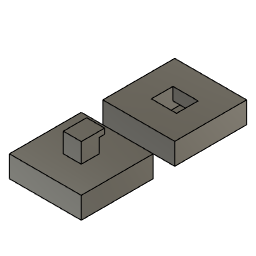
Latch cube 1 v2 (Autodesk Fusion 360 design; units mm, degrees)
Autodesk Fusion 360 part; units mm, degrees
sketch "Sketch1" plane through (0, 0, 0) normal (0, 0, 1) x (1, 0, 0) in component "Out put"
  line L0 (10, -10) -> (-10, -10)
  line L1 (-10, -10) -> (-10, 10)
  line L2 (-10, 10) -> (10, 10)
  line L3 (10, 10) -> (10, -10)
  line L4 (10, -10) -> (-10, 10) construction
  line L5 (-10, -10) -> (10, 10) construction
  dimension "d1" = 20
  dimension "d2" = 20
  constraint horizontal L0
  constraint perpendicular L0 L1
  constraint parallel L0 L2
  constraint parallel L1 L3
  constraint coincident L4 origin
  constraint coincident L5 origin
  measures "d1" distance of L1.end L2.end
  measures "d2" distance of L0.end L1.end
extrude "Extrude1" add sketch "Sketch1" along normal blind 6 makes body 1 in component "Out put"
sketch "Sketch2" plane through (0, 0, 6) normal (0, 0, 1) x (-1, 0, 0) in component "Out put"
  line L0 (-10, -10) -> (10, -10)
  line L1 (10, -10) -> (10, 10)
  line L2 (10, 10) -> (-10, 10)
  line L3 (-10, 10) -> (-10, -10)
  line L4 (-2.5, 2.5) -> (2.5, 2.5)
  line L5 (2.5, 2.5) -> (2.5, -2.5)
  line L6 (2.5, -2.5) -> (-2.5, -2.5)
  line L7 (-2.5, -2.5) -> (-2.5, 2.5)
  line L8 (-2.5, 2.5) -> (2.5, -2.5) construction
  line L9 (2.5, 2.5) -> (-2.5, -2.5) construction
  dimension "d5" = 5
  dimension "d6" = 5
  constraint horizontal L4
  constraint perpendicular L4 L5
  constraint parallel L4 L6
  constraint parallel L5 L7
  constraint coincident L8 origin
  constraint coincident L9 origin
  measures "d5" distance of L5.end L6.end
  measures "d6" distance of L4.end L5.end
extrude "Extrude2" add sketch "Sketch2" along normal blind 5.45 contours L4 L5 L6 L7 bodies 1 in component "Out put"
sketch "Sketch3" plane through (0, 2.5, 0) normal (0, 1, 0) x (-1, 0, 0) in component "Out put"
  line L0 (-2.5, 6) -> (2.5, 6)
  line L1 (2.5, 6) -> (2.5, 11.45)
  line L2 (2.5, 11.45) -> (-2.5, 11.45)
  line L3 (-2.5, 11.45) -> (-2.5, 6)
  line L4 (-2.5, 11.45) -> (2.5, 11.45)
  line L5 (2.5, 11.45) -> (2.5, 9.95)
  line L6 (2.5, 9.95) -> (-2.5, 9.95)
  line L7 (-2.5, 9.95) -> (-2.5, 11.45)
  dimension "d9" = 5
  dimension "d10" = 1.5
  constraint horizontal L4
  constraint vertical L5
  constraint horizontal L6
  constraint vertical L7
  constraint coincident L2.end L3.start
  measures "d9" distance of L2.end L1.end
  measures "d10" distance of L2.end L6.end
extrude "Extrude3" add sketch "Sketch3" along normal blind 1.5 contours L1 L2 L3 L4 L5 L6 L7 bodies 1 in component "Out put"
move_body "Move1" bodies 1 to x (1, 0, 0) y (0, 1, 0) z (0, 0, 1) at (0, -30, 0) in component "Out put"
sketch "Sketch1 (2)" plane through (0, 0, 0) normal (0, 0, 1) x (1, 0, 0) in component "Input"
  line L0 (-10, 10) -> (10, 10)
  line L1 (10, 10) -> (10, -10)
  line L2 (10, -10) -> (-10, -10)
  line L3 (-10, -10) -> (-10, 10)
  line L4 (-10, 10) -> (10, -10) construction
  line L5 (10, 10) -> (-10, -10) construction
  dimension "d13" = 20
  dimension "d14" = 20
  constraint horizontal L0
  constraint perpendicular L0 L1
  constraint parallel L0 L2
  constraint parallel L1 L3
  constraint coincident L4 origin
  constraint coincident L5 origin
  measures "d13" distance of L1.end L2.end
  measures "d14" distance of L0.end L1.end
extrude "Extrude1'" add sketch "Sketch1 (2)" along normal blind 6 separate body makes body 2 in component "Input"
sketch "Sketch3 (2)" plane through (0, 0, 6) normal (0, 0, 1) x (-1, 0, 0) in component "Input"
  line L0 (10, 10) -> (-10, 10)
  line L1 (-10, 10) -> (-10, -10)
  line L2 (-10, -10) -> (10, -10)
  line L3 (10, -10) -> (10, 10)
  line L4 (-3.5, 3) -> (3.5, 3)
  line L5 (3.5, 3) -> (3.5, -3)
  line L6 (3.5, -3) -> (-3.5, -3)
  line L7 (-3.5, -3) -> (-3.5, 3)
  line L8 (-3.5, 3) -> (3.5, -3) construction
  line L9 (3.5, 3) -> (-3.5, -3) construction
  dimension "d21" = 7
  dimension "d22" = 6
  constraint horizontal L4
  constraint perpendicular L4 L5
  constraint parallel L4 L6
  constraint parallel L5 L7
  constraint coincident L8 origin
  constraint coincident L9 origin
  measures "d21" distance of L5.end L6.end
  measures "d22" distance of L4.end L5.end
extrude "Extrude3'" cut sketch "Sketch3 (2)" against normal blind 5.5 contours L4 L5 L6 L7 bodies 2 in component "Input"
sketch "Sketch4" plane through (0, 3, 0) normal (0, -1, 0) x (1, 0, 0) in component "Input"
  line L0 (3.5, 6) -> (-3.5, 6)
  line L1 (-3.5, 6) -> (-3.5, 0.5)
  line L2 (-3.5, 0.5) -> (3.5, 0.5)
  line L3 (3.5, 0.5) -> (3.5, 6)
  line L4 (-3.5, 0.5) -> (3.5, 0.5)
  line L5 (3.5, 0.5) -> (3.5, 2.5)
  line L6 (3.5, 2.5) -> (-3.5, 2.5)
  line L7 (-3.5, 2.5) -> (-3.5, 0.5)
  dimension "d25" = 7
  dimension "d26" = 2
  constraint horizontal L4
  constraint vertical L5
  constraint horizontal L6
  constraint vertical L7
  constraint coincident L1.end L2.start
  measures "d25" distance of L1.end L2.end
  measures "d26" distance of L1.end L6.end
extrude "Extrude4" cut sketch "Sketch4" against normal blind 2 contours L1 L2 L3 L4 L5 L6 L7 bodies 2 in component "Input"
sketch "Sketch5" plane through (3.5, 0, 0) normal (-1, 0, 0) x (0, -1, 0) in component "Input"
  line L0 (3, 6) -> (-3, 6)
  line L1 (-3, 6) -> (-3, 2.5)
  line L2 (-3, 2.5) -> (-5, 2.5)
  line L3 (-5, 2.5) -> (-5, 0.5)
  line L4 (-5, 0.5) -> (3, 0.5)
  line L5 (3, 0.5) -> (3, 6)
  line L6 (-5, 0.5) -> (3, 0.5)
  line L7 (3, 0.5) -> (3, 2.5)
  line L8 (3, 2.5) -> (-5, 2.5)
  line L9 (-5, 2.5) -> (-5, 0.5)
  dimension "d29" = 8
  dimension "d30" = 2
  constraint horizontal L6
  constraint vertical L7
  constraint horizontal L8
  constraint vertical L9
  constraint coincident L3.end L4.start
  measures "d29" distance of L3.end L4.end
  measures "d30" distance of L3.end L2.end
extrude "Extrude5" cut sketch "Sketch5" against normal blind 2 contours L2 L3 L4 L5 L6 L7 L8 L9 bodies 2 in component "Input"
move_body "Move1'" bodies 2 to x (1, 0, 0) y (0, 1, 0) z (0, 0, 1) at (0, 13, 0) in component "Input"
component "Out put" placed x (1, 0, 0) y (0, 1, 0) z (0, 0, 1) at (0, 0, 0)
component "Input" placed x (1, 0, 0) y (0, 1, 0) z (0, 0, 1) at (0, 0, 0)
